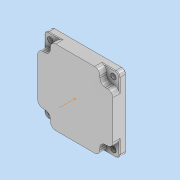
# Autodesk Inventor part: SERVO  KH56KM2U121 A
Saved by Autodesk Inventor 2021 (Build 250183000, 183)
## iProperties
Created: 2021-10-05
Part Number: SERVO  KH56KM2U121 A
Material: Generic
Document SubType Name: Modeling
Designer: 41601100
Density: 1 g/cm^3
Appearance: Default
Author: 41601100
Autodesk Inventor part; units mm, degrees
ref_plane "YZ Plane" through (0, 0, 0) normal (1, 0, 0) x (0, 1, 0)
ref_plane "XZ Plane" through (0, 0, 0) normal (0, 1, 0) x (-1, 0, 0)
ref_plane "XY Plane" through (0, 0, 0) normal (0, 0, 1) x (1, 0, 0)
sketch "Sketch1" plane through (0, 0, 0) normal (0, 0, 1) x (1, 0, 0)
  line L0 (28, 0) -> (28, 25)
  line L1 (25, 28) -> (-25, 28)
  line L2 (-28, 25) -> (-28, -25)
  line L3 (-25, -28) -> (25, -28)
  line L4 (28, -25) -> (28, 0)
  circle A0 centre (23.57, 23.57) radius 2
  circle A1 centre (23.57, -23.57) radius 2
  circle A2 centre (-23.57, -23.57) radius 2
  circle A3 centre (-23.57, 23.57) radius 2
  circle A4 centre (0, 0) radius 4.75
  circle A5 centre (0, 0) radius 15
  circle A6 centre (0, 0) radius 19.05
  arc A7 (-25, 28) -> (-28, 25) centre (-25, 25) ccw
  arc A8 (-28, -25) -> (-25, -28) centre (-25, -25) ccw
  arc A9 (25, -28) -> (28, -25) centre (25, -25) ccw
  arc A10 (28, 25) -> (25, 28) centre (25, 25) ccw
  circle A11 centre (0, 0) radius 3.15
  point P0 (28, 28)
  point P1 (-28, 28)
  point P2 (-28, -28)
  point P3 (28, -28)
  dimension "d1" = 28
  dimension "d2" = 56
  dimension "d3" = 56
  dimension "d4" = 56
  dimension "d6" = 4
  dimension "d7" = 4
  dimension "d8" = 4
  dimension "d9" = 4
  dimension "d10" = 9.5
  dimension "d11" = 30
  dimension "d12" = 38.1
  dimension "d13" = 3
  dimension "d25" = 6.3
  constraints: 12 centre point, 10 end point, 9 point on line, 8 point on circle, 8 tangent, 4 coincident, 3 equal radius, 2 perpendicular, 1 collinear
  measures "d1" distance of L0.start point (28, 28)
  measures "d2" distance of point (28, 28) point (-28, 28)
  measures "d3" distance of point (-28, 28) point (-28, -28)
  measures "d4" distance of point (-28, -28) point (28, -28)
  measures "d6" diameter of A0
  measures "d7" diameter of A1
  measures "d8" diameter of A2
  measures "d9" diameter of A3
  measures "d10" diameter of A4
  measures "d11" diameter of A5
  measures "d12" diameter of A6
  measures "d13" radius of A7
  measures "d25" diameter of A11
extrude "Extrusion1" add sketch "Sketch1" along normal blind 5 contours L4 A9 L3 A8 L2 A7 L1 A10 L0 | A4 | A5 | A6 | A11
extrude "Extrusion2" cut sketch "Sketch1" along normal blind 2 contours A4 | A6
sketch "Sketch2" plane through (0, 0, 5) normal (0, 0, 1) x (1, 0, 0)
  arc A0 (28, 25) -> (25, 28) centre (25, 25) ccw projected
  line L0 (25, 28) -> (-25, 28) projected
  arc A1 (-25, 28) -> (-28, 25) centre (-25, 25) ccw projected
  line L1 (-28, 25) -> (-28, -25) projected
  arc A2 (-28, -25) -> (-25, -28) centre (-25, -25) ccw projected
  line L2 (-25, -28) -> (25, -28) projected
  arc A3 (25, -28) -> (28, -25) centre (25, -25) ccw projected
  line L3 (28, -25) -> (28, 25) projected
  circle A4 centre (-23.57, 23.57) radius 2 projected
  circle A5 centre (-23.57, -23.57) radius 2 projected
  circle A6 centre (23.57, -23.57) radius 2 projected
  circle A7 centre (23.57, 23.57) radius 2 projected
  line L4 (-28, 0) -> (-28, 14.5)
  line L5 (-28, 25) -> (-28, -25) projected
  line L6 (-28, 0) -> (-28, -14.5)
  line L7 (25, 28) -> (-25, 28) projected
  line L8 (-25, -28) -> (25, -28) projected
  line L9 (-14.5, 28) -> (14.5, 28)
  line L10 (28, 14.5) -> (28, -14.5)
  line L11 (28, -25) -> (28, 25) projected
  line L12 (14.5, -28) -> (-14.5, -28)
  line L13 (-24, 18.5) -> (-22.5, 18.5)
  line L14 (22.5, 18.5) -> (24, 18.5)
  line L15 (-18.5, 24) -> (-18.5, 22.5)
  line L16 (-18.5, -22.5) -> (-18.5, -24)
  line L17 (18.5, 24) -> (18.5, 22.5)
  line L18 (18.5, -22.5) -> (18.5, -24)
  line L19 (-24, -18.5) -> (-22.5, -18.5)
  line L20 (22.5, -18.5) -> (24, -18.5)
  arc A8 (-14.5, 28) -> (-18.5, 24) centre (-14.5, 24) ccw
  arc A9 (-22.5, 18.5) -> (-18.5, 22.5) centre (-22.5, 22.5) ccw
  arc A10 (-24, 18.5) -> (-28, 14.5) centre (-24, 14.5) ccw
  arc A11 (-28, -14.5) -> (-24, -18.5) centre (-24, -14.5) ccw
  arc A12 (-18.5, -22.5) -> (-22.5, -18.5) centre (-22.5, -22.5) ccw
  arc A13 (-18.5, -24) -> (-14.5, -28) centre (-14.5, -24) ccw
  arc A14 (14.5, -28) -> (18.5, -24) centre (14.5, -24) ccw
  arc A15 (22.5, -18.5) -> (18.5, -22.5) centre (22.5, -22.5) ccw
  arc A16 (24, -18.5) -> (28, -14.5) centre (24, -14.5) ccw
  arc A17 (18.5, 24) -> (14.5, 28) centre (14.5, 24) ccw
  arc A18 (18.5, 22.5) -> (22.5, 18.5) centre (22.5, 22.5) ccw
  arc A19 (28, 14.5) -> (24, 18.5) centre (24, 14.5) ccw
  point P0 (0, 0)
  point P1 (-28, 18.5)
  point P2 (28, 18.5)
  point P3 (-28, -18.5)
  point P4 (28, -18.5)
  point P5 (18.5, 28)
  point P6 (18.5, -28)
  point P7 (-18.5, 28)
  point P8 (-18.5, -28)
  dimension "d18" = 18.5
  dimension "d19" = 18.5
  dimension "d22" = 4
  constraints: 26 end point, 24 point on circle, 24 tangent, 23 point on line, 12 centre point, 11 equal radius, 9 perpendicular, 2 collinear, 1 midpoint
  measures "d18" distance of L4.start point (-28, 18.5)
  measures "d19" distance of L4.start point (-28, -18.5)
  measures "d22" radius of A8
extrude "Extrusion3" add sketch "Sketch2" along normal blind 5 contours L3 A16 L20 A15 L18 A14 L2 A13 L16 A12 L19 A11 L1 A10 L13 A9 L15 A8 L0 A17 L17 A18 L14 A19
extrude "Extrusion4" add sketch "Sketch1" against normal blind 20.6 contours A11
sketch "Sketch3" plane through (0, 0, 10) normal (0, 0, 1) x (1, 0, 0)
  arc A0 (-24, 18.5) -> (-28, 14.5) centre (-24, 14.5) ccw projected
  line L0 (-28, 14.5) -> (-28, -14.5) projected
  arc A1 (-28, -14.5) -> (-24, -18.5) centre (-24, -14.5) ccw projected
  line L1 (-24, -18.5) -> (-22.5, -18.5) projected
  arc A2 (-18.5, -22.5) -> (-22.5, -18.5) centre (-22.5, -22.5) ccw projected
  line L2 (-18.5, -22.5) -> (-18.5, -24) projected
  arc A3 (-18.5, -24) -> (-14.5, -28) centre (-14.5, -24) ccw projected
  line L3 (-14.5, -28) -> (14.5, -28) projected
  arc A4 (14.5, -28) -> (18.5, -24) centre (14.5, -24) ccw projected
  line L4 (18.5, -24) -> (18.5, -22.5) projected
  arc A5 (22.5, -18.5) -> (18.5, -22.5) centre (22.5, -22.5) ccw projected
  line L5 (22.5, -18.5) -> (24, -18.5) projected
  arc A6 (24, -18.5) -> (28, -14.5) centre (24, -14.5) ccw projected
  line L6 (28, -14.5) -> (28, 14.5) projected
  arc A7 (28, 14.5) -> (24, 18.5) centre (24, 14.5) ccw projected
  line L7 (24, 18.5) -> (22.5, 18.5) projected
  arc A8 (18.5, 22.5) -> (22.5, 18.5) centre (22.5, 22.5) ccw projected
  line L8 (18.5, 22.5) -> (18.5, 24) projected
  arc A9 (18.5, 24) -> (14.5, 28) centre (14.5, 24) ccw projected
  line L9 (14.5, 28) -> (-14.5, 28) projected
  arc A10 (-14.5, 28) -> (-18.5, 24) centre (-14.5, 24) ccw projected
  line L10 (-18.5, 24) -> (-18.5, 22.5) projected
  arc A11 (-22.5, 18.5) -> (-18.5, 22.5) centre (-22.5, 22.5) ccw projected
  line L11 (-22.5, 18.5) -> (-24, 18.5) projected
  point P0 (0, 0)
extrude "Extrusion5" add sketch "Sketch1" against normal blind 1.6 contours A5
fillet "Fillet1" radius 0.5 24 edges at (27.1213, -27.1213, 0) (28, 0, 0) (27.1213, 27.1213, 0) (0, 28, 0) (-27.1213, 27.1213, 0) (-28, 0, 0) (-27.1213, -27.1213, 0) (0, -28, 0) (-19.05, 0, 0) (-15, 0, -1.6) (-3.15, 0, -20.6) (27.1213, 27.1213, 5) (19.75, 28, 5) (28, 19.75, 5) (-27.1213, 27.1213, 5) (-28, 19.75, 5) (-19.75, 28, 5) (-19.75, -28, 5) (-28, -19.75, 5) (-27.1213, -27.1213, 5) (27.1213, -27.1213, 5) (28, -19.75, 5) (19.75, -28, 5) (-4.75, 0, -1.6)
fillet "Fillet2" radius 0.1 8 edges at (21.57, -23.57, 0) (21.57, 23.57, 0) (-25.57, 23.57, 0) (-25.57, -23.57, 0) (-25.57, 23.57, 5) (21.57, 23.57, 5) (21.57, -23.57, 5) (-25.57, -23.57, 5)
sketch "Sketch4" plane through (0, 0, 0) normal (0, 0, -1) x (-1, 0, 0)
  circle A0 centre (23.57, 23.57) radius 2.1 projected
  circle A1 centre (-23.57, -23.57) radius 2.1 projected
  arc A2 (-27.5, -25) -> (-25, -27.5) centre (-25, -25) ccw projected
  line L0 (25, -27.5) -> (-25, -27.5) projected
  arc A3 (25, -27.5) -> (27.5, -25) centre (25, -25) ccw projected
  line L1 (27.5, 25) -> (27.5, -25) projected
  arc A4 (27.5, 25) -> (25, 27.5) centre (25, 25) ccw projected
  line L2 (-25, 27.5) -> (25, 27.5) projected
  arc A5 (-25, 27.5) -> (-27.5, 25) centre (-25, 25) ccw projected
  line L3 (-27.5, -25) -> (-27.5, 25) projected
  circle A6 centre (0, 0) radius 19.55 projected
  circle A7 centre (-23.57, 23.57) radius 2.1 projected
  circle A8 centre (23.57, -23.57) radius 2.1 projected
body "Solid1"
